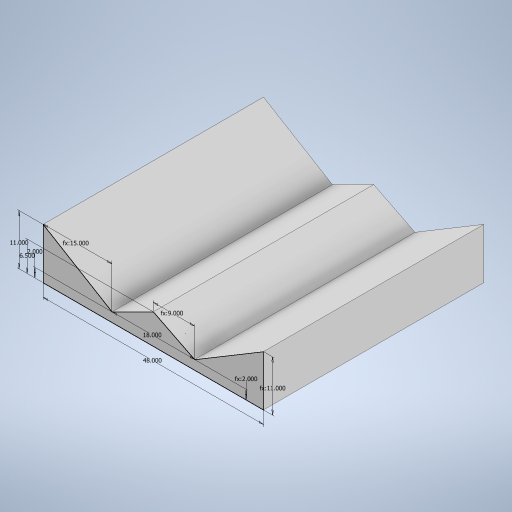
# Autodesk Inventor part: Drone Charging Base
Saved by Autodesk Inventor 2023 (Build 270158000, 158)
## iProperties
Created: 2022-12-15
Part Number: Drone Charging Base
Material: Generic
Document SubType Name: Modeling
Designer: chase
Density: 1 g/cm^3
Appearance: Default
Author: chase
Autodesk Inventor part; units mm, degrees
ref_plane "YZ Plane" through (0, 0, 0) normal (1, 0, 0) x (0, 1, 0)
ref_plane "XZ Plane" through (0, 0, 0) normal (0, 1, 0) x (-1, 0, 0)
ref_plane "XY Plane" through (0, 0, 0) normal (0, 0, 1) x (1, 0, 0)
sketch "Sketch1" plane through (0, 0, 0) normal (0, 0, 1) x (1, 0, 0)
  line L0 (0, 0) -> (1219.2, 0)
  line L1 (1219.2, 0) -> (1219.2, 279.4)
  line L2 (0, 279.4) -> (0, 0)
  line L3 (381, 50.8) -> (0, 279.4)
  line L4 (838.2, 50.8) -> (1219.2, 279.4)
  line L5 (330.2, 152.0857) -> (330.5143, 152.4)
  line L6 (787.7143, 152.4) -> (787.4, 152.4)
  line L7 (127, 152.4) -> (126.6857, 152.4)
  line L8 (381, 50.8) -> (609.6, 165.1)
  line L9 (838.2, 50.8) -> (609.6, 165.1)
  dimension "d37" = 165.1
  dimension "d39" = 457.2
  dimension "d40" = 1219.2
  dimension "d41" = 381
  dimension "d43" = 279.4
  dimension "d44" = 279.4
  dimension "d45" = 50.8
  dimension "d46" = 50.8
  dimension "d47" = 228.6
  constraints: 20 end point, 3 parallel, 1 horizontal, 1 perpendicular
  measures "d37" distance from line of L0 L8.end
  measures "d39" distance of L4.start L3.start
  measures "d40" distance of L0.start L0.end
  measures "d41" distance from line of L2 L3.start
  measures "d43" distance of L2.start L0.start
  measures "d44" distance of L0.end L1.end
  measures "d45" distance from line of L0 L3.start
  measures "d46" distance from line of L0 L4.start
  measures "d47" horizontal distance of L4.start L8.end
extrude "Extrusion3" add sketch "Sketch1" against normal blind 1219.2
body "Solid2"
